Autodesk Fusion 360 part; units mm, degrees
note: some values were not read from the file. Set by a fixed rule: which sketch regions a step uses.
(part 3 of 3)
sketch "Sketch9" plane through (0, 0, 26) normal (0, 0, 1) x (-1, 0, 0)
  arc A0 (-15, -36.168) -> (-14, -37.168) centre (-14, -36.168) ccw
  line L0 (-14, -37.168) -> (14, -37.168)
  arc A1 (14, -37.168) -> (15, -36.168) centre (14, -36.168) ccw
  line L1 (15, -36.168) -> (15, -29.9001)
  arc A2 (15, -29.9001) -> (14.5, -29.0341) centre (14, -29.9001) ccw
  line L2 (14.5, -29.0341) -> (11.5, -27.302)
  arc A3 (11, -26.436) -> (11.5, -27.302) centre (12, -26.436) ccw
  line L3 (11, -26.436) -> (11, 13.6823)
  arc A4 (11.5, 14.5484) -> (11, 13.6823) centre (12, 13.6823) ccw
  line L4 (11.5, 14.5484) -> (15.5, 16.8578)
  arc A5 (15.5, 16.8578) -> (16, 17.7238) centre (15, 17.7238) ccw
  line L5 (16, 17.7238) -> (16, 20.7956)
  arc A6 (16, 20.7956) -> (15.5, 21.6616) centre (15, 20.7956) ccw
  line L6 (15.5, 21.6616) -> (11.5, 23.971)
  arc A7 (11, 24.837) -> (11.5, 23.971) centre (12, 24.837) ccw
  line L7 (11, 24.837) -> (11, 57.116)
  arc A8 (11, 57.116) -> (10.342, 58.0557) centre (10, 57.116) ccw
  line L8 (10.342, 58.0557) -> (6.7055, 59.3792)
  arc A9 (6.7055, 59.3792) -> (6.0502, 59.4996) centre (6.0215, 57.4998) ccw
  arc A10 (6.0502, 59.4996) -> (3.3188, 58.2498) centre (6, 56) ccw
  line L9 (3.3188, 58.2498) -> (0.766, 55.2074)
  arc A11 (-0.766, 55.2074) -> (0.766, 55.2074) centre (0, 55.8502) ccw
  line L10 (-0.766, 55.2074) -> (-3.3188, 58.2498)
  arc A12 (-3.3188, 58.2498) -> (-6.0502, 59.4996) centre (-6, 56) ccw
  arc A13 (-6.0502, 59.4996) -> (-6.7055, 59.3792) centre (-6.0215, 57.4998) ccw
  line L11 (-6.7055, 59.3792) -> (-10.342, 58.0557)
  arc A14 (-10.342, 58.0557) -> (-11, 57.116) centre (-10, 57.116) ccw
  line L12 (-11, 57.116) -> (-11, 24.837)
  arc A15 (-11.5, 23.971) -> (-11, 24.837) centre (-12, 24.837) ccw
  line L13 (-11.5, 23.971) -> (-15.5, 21.6616)
  arc A16 (-15.5, 21.6616) -> (-16, 20.7956) centre (-15, 20.7956) ccw
  line L14 (-16, 20.7956) -> (-16, 17.7238)
  arc A17 (-16, 17.7238) -> (-15.5, 16.8578) centre (-15, 17.7238) ccw
  line L15 (-15.5, 16.8578) -> (-11.5, 14.5484)
  arc A18 (-11, 13.6823) -> (-11.5, 14.5484) centre (-12, 13.6823) ccw
  line L16 (-11, 13.6823) -> (-11, -26.436)
  arc A19 (-11.5, -27.302) -> (-11, -26.436) centre (-12, -26.436) ccw
  line L17 (-11.5, -27.302) -> (-14.5, -29.0341)
  arc A20 (-14.5, -29.0341) -> (-15, -29.9001) centre (-14, -29.9001) ccw
  line L18 (-15, -29.9001) -> (-15, -36.168)
  arc A21 (-11.1, -33.6647) -> (-11.4962, -32.018) centre (-8.5, -32.168) ccw
  line L19 (-11.1, -33.6647) -> (-11.1, -36.318)
  line L20 (-11.1, -36.318) -> (-13.9, -36.318)
  line L21 (-13.9, -36.318) -> (-13.9, -32.018)
  line L22 (-13.9, -32.018) -> (-11.4962, -32.018)
  circle A22 centre (6, 56) radius 3
  circle A23 centre (12.5, 19.2597) radius 3
  circle A24 centre (-6, 56) radius 3
  circle A25 centre (-12.5, 19.2597) radius 3
  arc A26 (11.4962, -32.018) -> (11.1, -33.6647) centre (8.5, -32.168) ccw
  line L23 (11.4962, -32.018) -> (13.9, -32.018)
  line L24 (13.9, -32.018) -> (13.9, -36.318)
  line L25 (13.9, -36.318) -> (11.1, -36.318)
  line L26 (11.1, -36.318) -> (11.1, -33.6647)
  line L27 (7, -22.168) -> (5.5, -22.168)
  line L28 (4.5, -21.168) -> (4.5, 11.832)
  line L29 (5.5, 12.832) -> (7, 12.832)
  line L30 (8, 11.832) -> (8, -21.168)
  line L31 (-7, -22.168) -> (-5.5, -22.168)
  line L32 (-4.5, -21.168) -> (-4.5, 11.832)
  line L33 (-5.5, 12.832) -> (-7, 12.832)
  line L34 (-8, 11.832) -> (-8, -21.168)
  arc A27 (4.5, -21.168) -> (5.5, -22.168) centre (5.5, -21.168) ccw
  arc A28 (7, -22.168) -> (8, -21.168) centre (7, -21.168) ccw
  arc A29 (8, 11.832) -> (7, 12.832) centre (7, 11.832) ccw
  arc A30 (5.5, 12.832) -> (4.5, 11.832) centre (5.5, 11.832) ccw
  arc A31 (-4.5, 11.832) -> (-5.5, 12.832) centre (-5.5, 11.832) ccw
  arc A32 (-7, 12.832) -> (-8, 11.832) centre (-7, 11.832) ccw
  arc A33 (-8, -21.168) -> (-7, -22.168) centre (-7, -21.168) ccw
  arc A34 (-5.5, -22.168) -> (-4.5, -21.168) centre (-5.5, -21.168) ccw
  point P0 (8, -22.168)
  point P1 (4.5, -22.168)
  point P2 (8, 12.832)
  point P3 (-8, -22.168)
  point P4 (-4.5, -22.168)
  point P5 (-8, 12.832)
  dimension "d375" = 3.5
  dimension "d376" = 35
  dimension "d377" = 3.5
  dimension "d378" = 35
  dimension "d379" = 3
  dimension "d380" = 3
  dimension "d381" = 10
  dimension "d382" = 10
  dimension "d383" = 1
  constraint horizontal L27
  constraint vertical L28
  constraint horizontal L29
  constraint vertical L30
  constraint horizontal L31
  constraint vertical L32
  constraint horizontal L33
  constraint vertical L34
  constraint coincident P1 L27
  constraint coincident P1 L28
  constraint tangent L27 A27
  constraint tangent L28 A27
  constraint coincident P0 L27
  constraint coincident P0 L30
  constraint tangent L27 A28
  constraint tangent L30 A28
  constraint equal A27 A28
  constraint coincident P2 L29
  constraint coincident P2 L30
  constraint tangent L29 A29
  constraint tangent L30 A29
  constraint equal A27 A29
  constraint tangent L28 A30
  constraint tangent L29 A30
  constraint equal A27 A30
  constraint tangent L32 A31
  constraint tangent L33 A31
  constraint equal A27 A31
  constraint coincident P5 L33
  constraint coincident P5 L34
  constraint tangent L33 A32
  constraint tangent L34 A32
  constraint equal A27 A32
  constraint coincident P3 L31
  constraint coincident P3 L34
  constraint tangent L31 A33
  constraint tangent L34 A33
  constraint equal A27 A33
  constraint coincident P4 L31
  constraint coincident P4 L32
  constraint tangent L31 A34
  constraint tangent L32 A34
  constraint equal A27 A34
  measures "d375" distance of P0 P1
  measures "d376" distance of P0 P2
  measures "d377" distance of P3 P4
  measures "d378" distance of P3 P5
  measures "d379" distance of L3 L30
  measures "d380" distance of L16 L34
  measures "d381" distance of A26.centre L27
  measures "d382" distance of A21.centre L31
  measures "d383" radius of A27
extrude "Extrude18" cut sketch "Sketch9" against normal blind 2 contours L27 L28 L29 L30 A27 A28 A29 A30 | L31 L32 L33 L34 A31 A32 A33 A34 bodies 2
sketch "Sketch10" plane through (11.25, 0, 0) normal (-1, 0, 0) x (0, -1, 0)
  circle A0 centre (-47.1705, 15.3) radius 1
  spline S0 degree 2 poles (-32.168, 25.75) (-32.7415, 25.75) (-33.367, 26) knots 0.122474 0.122474 0.122474 0.244949 0.244949 0.244949 weights 1.045455 1.045455 1
  line L0 (-33.367, 26) -> (-36.168, 26)
  line L1 (-36.168, 26) -> (-36.168, 24)
  line L2 (-36.168, 24) -> (-37.168, 24)
  line L3 (-37.168, 24) -> (-53.2322, 29.8469)
  arc A1 (-53.2322, 29.8469) -> (-54.4692, 29.8895) centre (-53.9162, 27.9675) ccw
  line L4 (-54.4692, 29.8895) -> (-61.0301, 28.0017)
  arc A2 (-61.0301, 28.0017) -> (-62.3565, 26.7637) centre (-60.4771, 26.0797) ccw
  line L5 (-62.3565, 26.7637) -> (-66.646, 14.9783)
  arc A3 (-66.646, 14.9783) -> (-66.4049, 13.1472) centre (-64.7666, 14.2943) ccw
  line L6 (-66.4049, 13.1472) -> (-60.5972, 4.8528)
  arc A4 (-60.5972, 4.8528) -> (-58.9589, 4) centre (-58.9589, 6) ccw
  line L7 (-58.9589, 4) -> (-54.9589, 4)
  line L8 (-54.9589, 4) -> (-54.9589, 0)
  line L9 (-54.9589, 0) -> (-43.3899, 0)
  line L10 (-43.3899, 0) -> (-43.3899, 4)
  line L11 (-43.3899, 4) -> (-42.3899, 4)
  arc A5 (-42.3899, 4) -> (-40.9757, 4.5858) centre (-42.3899, 6) ccw
  line L12 (-40.9757, 4.5858) -> (-36.4293, 9.1322)
  arc A6 (-36.4293, 9.1322) -> (-35.9116, 10.0288) centre (-37.8435, 10.5464) ccw
  line L13 (-35.9116, 10.0288) -> (-32.168, 24)
  line L14 (-32.168, 24) -> (-32.168, 25.75)
  arc A7 (-50.4705, 8.5) -> (-49.4705, 7.5) centre (-49.4705, 8.5) ccw
  line L15 (-50.4705, 8.5) -> (-50.4705, 11.3223)
  arc A8 (-49.4608, 12.3222) -> (-50.4705, 11.3223) centre (-49.4705, 11.3223) ccw
  line L16 (-49.4608, 12.3222) -> (-47.1998, 12.3001)
  arc A9 (-47.1998, 12.3001) -> (-47.1705, 18.3) centre (-47.1705, 15.3) ccw
  line L17 (-47.1705, 18.3) -> (-49.4705, 18.3)
  arc A10 (-50.4705, 19.3) -> (-49.4705, 18.3) centre (-49.4705, 19.3) ccw
  line L18 (-50.4705, 19.3) -> (-50.4705, 23.6889)
  arc A11 (-49.1285, 24.6286) -> (-50.4705, 23.6889) centre (-49.4705, 23.6889) ccw
  line L19 (-49.1285, 24.6286) -> (-38.4432, 20.7395)
  arc A12 (-37.7852, 19.7998) -> (-38.4432, 20.7395) centre (-38.7852, 19.7998) ccw
  line L20 (-37.7852, 19.7998) -> (-37.7852, 16.6911)
  arc A13 (-37.8193, 16.4323) -> (-37.7852, 16.6911) centre (-38.7852, 16.6911) ccw
  line L21 (-37.8193, 16.4323) -> (-39.119, 11.5817)
  arc A14 (-39.3778, 11.1334) -> (-39.119, 11.5817) centre (-40.0849, 11.8405) ccw
  line L22 (-39.3778, 11.1334) -> (-42.7183, 7.7929)
  arc A15 (-43.4254, 7.5) -> (-42.7183, 7.7929) centre (-43.4254, 8.5) ccw
  line L23 (-43.4254, 7.5) -> (-49.4705, 7.5)
  arc A16 (-62.912, 15.0042) -> (-62.7914, 14.0886) centre (-61.9723, 14.6622) ccw
  line L24 (-62.912, 15.0042) -> (-59.5027, 24.371)
  arc A17 (-58.8395, 24.99) -> (-59.5027, 24.371) centre (-58.563, 24.029) ccw
  line L25 (-58.8395, 24.99) -> (-55.247, 26.0237)
  arc A18 (-53.9705, 25.0627) -> (-55.247, 26.0237) centre (-54.9705, 25.0627) ccw
  line L26 (-53.9705, 25.0627) -> (-53.9705, 8.5)
  arc A19 (-54.9705, 7.5) -> (-53.9705, 8.5) centre (-54.9705, 8.5) ccw
  line L27 (-54.9705, 7.5) -> (-57.6574, 7.5)
  arc A20 (-58.4766, 7.9264) -> (-57.6574, 7.5) centre (-57.6574, 8.5) ccw
  line L28 (-58.4766, 7.9264) -> (-62.7914, 14.0886)
  circle A21 centre (-47.1705, 15.3) radius 3
  constraint concentric A0 A21
extrude "Extrude19" add sketch "Sketch10" along normal blind 1.75 contours A9 A21 bodies 4
extrude "Extrude20" add sketch "Sketch10" against normal blind 1.75 from surface at 22.5 contours A9 A21 bodies 3
equation "d120 = 3\""
equation "d121 = 3\""
equation "d122 = 3\""
equation "d123 = 3\""
equation "d276 = 180 deg - 30 deg"
equation "d277 = 180 deg - 30 deg"
equation "d356 = 24.00 mm + ( 2 mm - 1.425 mm )"
named bodies: "bottomFrame", "topFrame", "leftCameraFrame", "rightCameraFrame"
